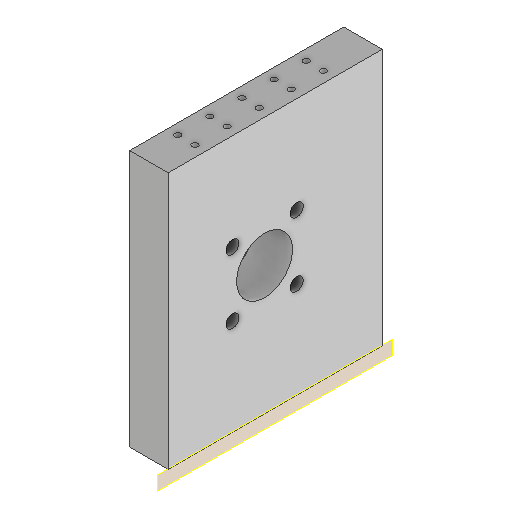
# Autodesk Inventor part: OpenFrameAdapter_2
Saved by Autodesk Inventor 2024.1 (Build 281209000, 209)
## iProperties
Created: 2024-06-05
Part Number: OpenFrameAdapter_2
Material: Generisch
Document SubType Name: Modeling
Designer: diederichbenedict
Density: 1 g/cm^3
Appearance: Vorgabe
Author: diederichbenedict
Autodesk Inventor part; units mm, degrees
ref_plane "YZ Plane" through (0, 0, 0) normal (1, 0, 0) x (0, 1, 0)
ref_plane "XZ Plane" through (0, 0, 0) normal (0, 1, 0) x (-1, 0, 0)
ref_plane "XY Plane" through (0, 0, 0) normal (0, 0, 1) x (1, 0, 0)
ref_plane "Arbeitsebene1" through (302.488, 50, 0) normal (1, 0, 0) x (0, -1, 0)
sketch "Skizze1" plane through (302.488, 50, 0) normal (1, 0, 0) x (0, -1, 0)
  line L0 (100, -120) -> (0, -120) projected
  line L1 (0, 0) -> (100, 0) projected
  line L2 (100, -120) -> (0, -120)
  line L3 (0, -120) -> (0, 0)
  line L4 (0, 0) -> (100, 0)
  line L5 (100, 0) -> (100, -120)
  circle A0 centre (55, -60) radius 13.0556 projected
  point P0 (50, 0)
  constraints: 8 end point, 2 parallel, 1 horizontal, 1 perpendicular
extrude "Extrusion1" add sketch "Skizze1" against normal blind 18
sketch "Skizze2" plane through (302.488, -50, 0) normal (0, 0, -1) x (-1, 0, 0)
  circle A0 centre (186.5, 89.5) radius 1.5 projected
  circle A1 centre (100.8, 89.5) radius 1.5 projected
  circle A2 centre (139.4003, 16.8597) radius 1.55 projected
  line L0 (398.9827, 14) -> (394.9827, 14) projected
  line L1 (394.9827, 14) -> (394.9827, 79) projected
  line L2 (394.9827, 79) -> (398.9827, 79) projected
  line L3 (398.9827, 79) -> (398.9827, 14) projected
  line L4 (252.25, 9) -> (252.25, 11.4) projected
  line L5 (252.25, 11.4) -> (257.75, 11.4) projected
  line L6 (257.75, 11.4) -> (257.75, 9) projected
  line L7 (257.75, 9) -> (252.25, 9) projected
  line L8 (457.75, 11.4) -> (457.75, 9) projected
  line L9 (457.75, 9) -> (452.25, 9) projected
  line L10 (452.25, 9) -> (452.25, 11.4) projected
  line L11 (452.25, 11.4) -> (457.75, 11.4) projected
  line L12 (57.75, 9) -> (52.25, 9) projected
  line L13 (52.25, 9) -> (52.25, 11.4) projected
  line L14 (52.25, 11.4) -> (57.75, 11.4) projected
  line L15 (57.75, 11.4) -> (57.75, 9) projected
  line L16 (352.25, 9) -> (352.25, 11.4) projected
  line L17 (352.25, 11.4) -> (357.75, 11.4) projected
  line L18 (357.75, 11.4) -> (357.75, 9) projected
  line L19 (357.75, 9) -> (352.25, 9) projected
  line L20 (157.75, 9) -> (152.25, 9) projected
  line L21 (152.25, 9) -> (152.25, 11.4) projected
  line L22 (152.25, 11.4) -> (157.75, 11.4) projected
  line L23 (157.75, 11.4) -> (157.75, 9) projected
  line L24 (257.75, 91) -> (257.75, 88.6) projected
  line L25 (257.75, 88.6) -> (252.25, 88.6) projected
  line L26 (252.25, 88.6) -> (252.25, 91) projected
  line L27 (252.25, 91) -> (257.75, 91) projected
  line L28 (157.75, 91) -> (157.75, 88.6) projected
  line L29 (157.75, 88.6) -> (152.25, 88.6) projected
  line L30 (152.25, 88.6) -> (152.25, 91) projected
  line L31 (152.25, 91) -> (157.75, 91) projected
  line L32 (357.75, 91) -> (357.75, 88.6) projected
  line L33 (357.75, 88.6) -> (352.25, 88.6) projected
  line L34 (352.25, 88.6) -> (352.25, 91) projected
  line L35 (352.25, 91) -> (357.75, 91) projected
  line L36 (57.75, 91) -> (57.75, 88.6) projected
  line L37 (57.75, 88.6) -> (52.25, 88.6) projected
  line L38 (52.25, 88.6) -> (52.25, 91) projected
  line L39 (52.25, 91) -> (57.75, 91) projected
  line L40 (452.25, 88.6) -> (452.25, 91) projected
  line L41 (452.25, 91) -> (457.75, 91) projected
  line L42 (457.75, 91) -> (457.75, 88.6) projected
  line L43 (457.75, 88.6) -> (452.25, 88.6) projected
  line L44 (449.9, 0) -> (449.9, 6) projected
  line L45 (449.9, 6) -> (460.1, 6) projected
  line L46 (460.1, 6) -> (460.1, 0) projected
  line L47 (460.1, 0) -> (490, 0) projected
  line L48 (490, 0) -> (490, 94) projected
  line L49 (490, 94) -> (470, 94) projected
  line L50 (470, 94) -> (470, 100) projected
  line L51 (470, 100) -> (460.1, 100) projected
  line L52 (460.1, 100) -> (460.1, 94) projected
  line L53 (460.1, 94) -> (449.9, 94) projected
  line L54 (449.9, 94) -> (449.9, 100) projected
  line L55 (449.9, 100) -> (440.1, 100) projected
  line L56 (440.1, 100) -> (440.1, 94) projected
  line L57 (440.1, 94) -> (429.9, 94) projected
  line L58 (429.9, 94) -> (429.9, 100) projected
  line L59 (429.9, 100) -> (420.1, 100) projected
  line L60 (420.1, 100) -> (420.1, 94) projected
  line L61 (420.1, 94) -> (409.9, 94) projected
  line L62 (409.9, 94) -> (409.9, 100) projected
  line L63 (409.9, 100) -> (400.1, 100) projected
  line L64 (400.1, 100) -> (400.1, 94) projected
  line L65 (400.1, 94) -> (389.9, 94) projected
  line L66 (389.9, 94) -> (389.9, 100) projected
  line L67 (389.9, 100) -> (380.1, 100) projected
  line L68 (380.1, 100) -> (380.1, 94) projected
  line L69 (380.1, 94) -> (369.9, 94) projected
  line L70 (369.9, 94) -> (369.9, 100) projected
  line L71 (369.9, 100) -> (360.1, 100) projected
  line L72 (360.1, 100) -> (360.1, 94) projected
  line L73 (360.1, 94) -> (349.9, 94) projected
  line L74 (349.9, 94) -> (349.9, 100) projected
  line L75 (349.9, 100) -> (340.1, 100) projected
  line L76 (340.1, 100) -> (340.1, 94) projected
  line L77 (340.1, 94) -> (329.9, 94) projected
  line L78 (329.9, 94) -> (329.9, 100) projected
  line L79 (329.9, 100) -> (320.1, 100) projected
  line L80 (320.1, 100) -> (320.1, 94) projected
  line L81 (320.1, 94) -> (309.9, 94) projected
  line L82 (309.9, 94) -> (309.9, 100) projected
  line L83 (309.9, 100) -> (300.1, 100) projected
  line L84 (300.1, 100) -> (300.1, 94) projected
  line L85 (300.1, 94) -> (289.9, 94) projected
  line L86 (289.9, 94) -> (289.9, 100) projected
  line L87 (289.9, 100) -> (280.1, 100) projected
  line L88 (280.1, 100) -> (280.1, 94) projected
  line L89 (280.1, 94) -> (269.9, 94) projected
  line L90 (269.9, 94) -> (269.9, 100) projected
  line L91 (269.9, 100) -> (260.1, 100) projected
  line L92 (260.1, 100) -> (260.1, 94) projected
  line L93 (260.1, 94) -> (249.9, 94) projected
  line L94 (249.9, 94) -> (249.9, 100) projected
  line L95 (249.9, 100) -> (240.1, 100) projected
  line L96 (240.1, 100) -> (240.1, 94) projected
  line L97 (240.1, 94) -> (229.9, 94) projected
  line L98 (229.9, 94) -> (229.9, 100) projected
  line L99 (229.9, 100) -> (220.1, 100) projected
  line L100 (220.1, 100) -> (220.1, 94) projected
  line L101 (220.1, 94) -> (209.9, 94) projected
  line L102 (209.9, 94) -> (209.9, 100) projected
  line L103 (209.9, 100) -> (200.1, 100) projected
  line L104 (200.1, 100) -> (200.1, 94) projected
  line L105 (200.1, 94) -> (189.9, 94) projected
  line L106 (189.9, 94) -> (189.9, 100) projected
  line L107 (189.9, 100) -> (180.1, 100) projected
  line L108 (180.1, 100) -> (180.1, 94) projected
  line L109 (180.1, 94) -> (169.9, 94) projected
  line L110 (169.9, 94) -> (169.9, 100) projected
  line L111 (169.9, 100) -> (160.1, 100) projected
  line L112 (160.1, 100) -> (160.1, 94) projected
  line L113 (160.1, 94) -> (149.9, 94) projected
  line L114 (149.9, 94) -> (149.9, 100) projected
  line L115 (149.9, 100) -> (140.1, 100) projected
  line L116 (140.1, 100) -> (140.1, 94) projected
  line L117 (140.1, 94) -> (129.9, 94) projected
  line L118 (129.9, 94) -> (129.9, 100) projected
  line L119 (129.9, 100) -> (120.1, 100) projected
  line L120 (120.1, 100) -> (120.1, 94) projected
  line L121 (120.1, 94) -> (109.9, 94) projected
  line L122 (109.9, 94) -> (109.9, 100) projected
  line L123 (109.9, 100) -> (100.1, 100) projected
  line L124 (100.1, 100) -> (100.1, 94) projected
  line L125 (100.1, 94) -> (89.9, 94) projected
  line L126 (89.9, 94) -> (89.9, 100) projected
  line L127 (89.9, 100) -> (80.1, 100) projected
  line L128 (80.1, 100) -> (80.1, 94) projected
  line L129 (80.1, 94) -> (69.9, 94) projected
  line L130 (69.9, 94) -> (69.9, 100) projected
  line L131 (69.9, 100) -> (60.1, 100) projected
  line L132 (60.1, 100) -> (60.1, 94) projected
  line L133 (60.1, 94) -> (49.9, 94) projected
  line L134 (49.9, 94) -> (49.9, 100) projected
  line L135 (49.9, 100) -> (0, 100) projected
  line L136 (0, 100) -> (0, 0) projected
  line L137 (0, 0) -> (49.9, 0) projected
  line L138 (49.9, 0) -> (49.9, 6) projected
  line L139 (49.9, 6) -> (60.1, 6) projected
  line L140 (60.1, 6) -> (60.1, 0) projected
  line L141 (60.1, 0) -> (69.9, 0) projected
  line L142 (69.9, 0) -> (69.9, 6) projected
  line L143 (69.9, 6) -> (80.1, 6) projected
  line L144 (80.1, 6) -> (80.1, 0) projected
  line L145 (80.1, 0) -> (89.9, 0) projected
  line L146 (89.9, 0) -> (89.9, 6) projected
  line L147 (89.9, 6) -> (100.1, 6) projected
  line L148 (100.1, 6) -> (100.1, 0) projected
  line L149 (100.1, 0) -> (109.9, 0) projected
  line L150 (109.9, 0) -> (109.9, 6) projected
  line L151 (109.9, 6) -> (120.1, 6) projected
  line L152 (120.1, 6) -> (120.1, 0) projected
  line L153 (120.1, 0) -> (129.9, 0) projected
  line L154 (129.9, 0) -> (129.9, 6) projected
  line L155 (129.9, 6) -> (140.1, 6) projected
  line L156 (140.1, 6) -> (140.1, 0) projected
  line L157 (140.1, 0) -> (149.9, 0) projected
  line L158 (149.9, 0) -> (149.9, 6) projected
  line L159 (149.9, 6) -> (160.1, 6) projected
  line L160 (160.1, 6) -> (160.1, 0) projected
  line L161 (160.1, 0) -> (169.9, 0) projected
  line L162 (169.9, 0) -> (169.9, 6) projected
  line L163 (169.9, 6) -> (180.1, 6) projected
  line L164 (180.1, 6) -> (180.1, 0) projected
  line L165 (180.1, 0) -> (189.9, 0) projected
  line L166 (189.9, 0) -> (189.9, 6) projected
  line L167 (189.9, 6) -> (200.1, 6) projected
  line L168 (200.1, 6) -> (200.1, 0) projected
  line L169 (200.1, 0) -> (209.9, 0) projected
  line L170 (209.9, 0) -> (209.9, 6) projected
  line L171 (209.9, 6) -> (220.1, 6) projected
  line L172 (220.1, 6) -> (220.1, 0) projected
  line L173 (220.1, 0) -> (229.9, 0) projected
  line L174 (229.9, 0) -> (229.9, 6) projected
  line L175 (229.9, 6) -> (240.1, 6) projected
  line L176 (240.1, 6) -> (240.1, 0) projected
  line L177 (240.1, 0) -> (249.9, 0) projected
  line L178 (249.9, 0) -> (249.9, 6) projected
  line L179 (249.9, 6) -> (260.1, 6) projected
  line L180 (260.1, 6) -> (260.1, 0) projected
  line L181 (260.1, 0) -> (269.9, 0) projected
  line L182 (269.9, 0) -> (269.9, 6) projected
  line L183 (269.9, 6) -> (280.1, 6) projected
  line L184 (280.1, 6) -> (280.1, 0) projected
  line L185 (280.1, 0) -> (289.9, 0) projected
  line L186 (289.9, 0) -> (289.9, 6) projected
  line L187 (289.9, 6) -> (300.1, 6) projected
  line L188 (300.1, 6) -> (300.1, 0) projected
  line L189 (300.1, 0) -> (309.9, 0) projected
  line L190 (309.9, 0) -> (309.9, 6) projected
  line L191 (309.9, 6) -> (320.1, 6) projected
  line L192 (320.1, 6) -> (320.1, 0) projected
  line L193 (320.1, 0) -> (329.9, 0) projected
  line L194 (329.9, 0) -> (329.9, 6) projected
  line L195 (329.9, 6) -> (340.1, 6) projected
  line L196 (340.1, 6) -> (340.1, 0) projected
  line L197 (340.1, 0) -> (349.9, 0) projected
  line L198 (349.9, 0) -> (349.9, 6) projected
  line L199 (349.9, 6) -> (360.1, 6) projected
  line L200 (360.1, 6) -> (360.1, 0) projected
  line L201 (360.1, 0) -> (369.9, 0) projected
  line L202 (369.9, 0) -> (369.9, 6) projected
  line L203 (369.9, 6) -> (380.1, 6) projected
  line L204 (380.1, 6) -> (380.1, 0) projected
  line L205 (380.1, 0) -> (389.9, 0) projected
  line L206 (389.9, 0) -> (389.9, 6) projected
  line L207 (389.9, 6) -> (400.1, 6) projected
  line L208 (400.1, 6) -> (400.1, 0) projected
  line L209 (400.1, 0) -> (409.9, 0) projected
  line L210 (409.9, 0) -> (409.9, 6) projected
  line L211 (409.9, 6) -> (420.1, 6) projected
  line L212 (420.1, 6) -> (420.1, 0) projected
  line L213 (420.1, 0) -> (429.9, 0) projected
  line L214 (429.9, 0) -> (429.9, 6) projected
  line L215 (429.9, 6) -> (440.1, 6) projected
  line L216 (440.1, 6) -> (440.1, 0) projected
  line L217 (440.1, 0) -> (449.9, 0) projected
  circle A3 centre (5, 47.5) radius 1.6 projected
  circle A4 centre (5, 62.5) radius 1.6 projected
  circle A5 centre (5, 32.5) radius 1.6 projected
  circle A6 centre (5, 77.5) radius 1.6 projected
  circle A7 centre (5, 17.5) radius 1.6 projected
  point P0 (302.488, 50)
hole "Bohrung1" at (297.488, -32.5, 0) at (297.488, -17.5, 0) at (297.488, -2.5, 0) at (297.488, 12.5, 0) at (297.488, 27.5, 0) direction (0, 0, 1) diameter 2.8 depth 14 tip angle 118
sketch "Skizze3" plane through (302.488, -50, 120) normal (0, 0, 1) x (1, 0, 0)
  circle A0 centre (-13.0375, 47.5) radius 1.6 projected
  circle A1 centre (-13.0375, 62.5) radius 1.6 projected
  circle A2 centre (-13.0375, 32.5) radius 1.6 projected
  circle A3 centre (-13.0375, 77.5) radius 1.6 projected
  circle A4 centre (-13.0375, 17.5) radius 1.6 projected
  line L0 (-97.75, 88.6) -> (-97.75, 91) projected
  line L1 (-97.75, 91) -> (-92.25, 91) projected
  line L2 (-92.25, 91) -> (-92.25, 88.6) projected
  line L3 (-92.25, 88.6) -> (-97.75, 88.6) projected
  line L4 (-57.75, 88.6) -> (-57.75, 91) projected
  line L5 (-57.75, 91) -> (-52.25, 91) projected
  line L6 (-52.25, 91) -> (-52.25, 88.6) projected
  line L7 (-52.25, 88.6) -> (-57.75, 88.6) projected
  line L8 (-100.2875, 11.4) -> (-100.2875, 9) projected
  line L9 (-100.2875, 9) -> (-105.7875, 9) projected
  line L10 (-105.7875, 9) -> (-105.7875, 11.4) projected
  line L11 (-105.7875, 11.4) -> (-100.2875, 11.4) projected
  line L12 (-25.7875, 9) -> (-25.7875, 11.4) projected
  line L13 (-25.7875, 11.4) -> (-20.2875, 11.4) projected
  line L14 (-20.2875, 11.4) -> (-20.2875, 9) projected
  line L15 (-20.2875, 9) -> (-25.7875, 9) projected
  line L16 (-123.0375, 8) -> (-122.8375, 8) projected
  line L17 (-122.8375, 8) -> (-122.8375, 6) projected
  line L18 (-123.0375, 6) -> (-123.0375, 3.8071) projected
  line L19 (-120.1, 6) -> (-109.9, 6) projected
  line L20 (-109.9, 6) -> (-117.9375, 0) projected
  line L21 (-117.9375, 0) -> (-108.1375, 0) projected
  line L22 (-108.1375, 0) -> (-100.1, 6) projected
  line L23 (-100.1, 6) -> (-89.9, 6) projected
  line L24 (-89.9, 6) -> (-97.9375, 0) projected
  line L25 (-97.9375, 0) -> (-88.1375, 0) projected
  line L26 (-88.1375, 0) -> (-80.1, 6) projected
  line L27 (-80.1, 6) -> (-69.9, 6) projected
  line L28 (-69.9, 6) -> (-77.9375, 0) projected
  line L29 (-77.9375, 0) -> (-68.1375, 0) projected
  line L30 (-68.1375, 0) -> (-60.1, 6) projected
  line L31 (-60.1, 6) -> (-49.9, 6) projected
  line L32 (-49.9, 6) -> (-57.9375, 0) projected
  line L33 (-57.9375, 0) -> (-48.1375, 0) projected
  line L34 (-48.1375, 0) -> (-40.1, 6) projected
  line L35 (-40.1, 6) -> (-29.9, 6) projected
  line L36 (-29.9, 6) -> (-37.9375, 0) projected
  line L37 (-37.9375, 0) -> (-28.1375, 0) projected
  line L38 (-28.1375, 0) -> (-20.1, 6) projected
  line L39 (-20.1, 6) -> (-9.9, 6) projected
  line L40 (-9.9, 6) -> (-17.9375, 0) projected
  line L41 (-17.9375, 0) -> (-8.0375, 0) projected
  line L42 (-49.9, 100) -> (-49.9, 94) projected
  line L43 (-49.9, 94) -> (-60.1, 94) projected
  line L44 (-60.1, 94) -> (-60.1, 100) projected
  line L45 (-69.9, 100) -> (-69.9, 94) projected
  line L46 (-69.9, 94) -> (-80.1, 94) projected
  line L47 (-80.1, 94) -> (-80.1, 100) projected
  line L48 (-89.9, 100) -> (-89.9, 94) projected
  line L49 (-89.9, 94) -> (-100.1, 94) projected
  line L50 (-100.1, 94) -> (-100.1, 100) projected
  line L51 (-110, 100) -> (-110, 94) projected
  line L52 (-110, 94) -> (-115, 94) projected
  circle A5 centre (-5, 77.5) radius 1.4 projected
  circle A6 centre (-5, 62.5) radius 1.4 projected
  circle A7 centre (-5, 47.5) radius 1.4 projected
  circle A8 centre (-5, 32.5) radius 1.4 projected
  circle A9 centre (-5, 17.5) radius 1.4 projected
  line L53 (0, 0) -> (0, 100) projected
  line L54 (0, 0) -> (-18, 0) projected
  line L55 (-18, 100) -> (-18, 0) projected
  line L56 (0, 100) -> (-18, 100) projected
  line L57 (-122.8375, 6) -> (-123.0375, 6) projected
  line L58 (-123.0375, 3.8071) -> (-120.1, 6) projected
  line L59 (-8.0375, 0) -> (-8.0375, 100) projected
  line L60 (-8.0375, 100) -> (-49.9, 100) projected
  line L61 (-60.1, 100) -> (-69.9, 100) projected
  line L62 (-80.1, 100) -> (-89.9, 100) projected
  line L63 (-100.1, 100) -> (-110, 100) projected
  line L64 (-115, 94) -> (-115, 100) projected
  line L65 (-115, 100) -> (-123.0375, 100) projected
  line L66 (-123.0375, 100) -> (-123.0375, 8) projected
  point P0 (-302.488, 50)
hole "Bohrung2" at (289.4504, 27.5, 120) at (289.4504, 12.5, 120) at (289.4504, -2.5, 120) at (289.4504, -17.5, 120) at (289.4504, -32.5, 120) at (297.488, -32.5, 120) at (297.488, -17.5, 120) at (297.488, -2.5, 120) at (297.488, 12.5, 120) at (297.488, 27.5, 120) direction (0, 0, -1) diameter 2.8 depth 14 tip angle 118
sketch "Skizze4" plane through (284.488, 50, 0) normal (-1, 0, 0) x (0, 0, 1)
  line L0 (39.934, -37.0712) -> (39.934, -72.9288) projected
  line L1 (39.934, -72.9288) -> (42.0712, -75.066) projected
  line L2 (42.0712, -75.066) -> (77.9288, -75.066) projected
  line L3 (77.9288, -75.066) -> (80.066, -72.9288) projected
  line L4 (80.066, -72.9288) -> (80.066, -37.0712) projected
  line L5 (80.066, -37.0712) -> (77.9288, -34.934) projected
  line L6 (77.9288, -34.934) -> (42.0712, -34.934) projected
  line L7 (42.0712, -34.934) -> (39.934, -37.0712) projected
  circle A0 centre (75, -70) radius 3.2639 projected
  circle A1 centre (45, -70) radius 3.2639 projected
  circle A2 centre (75, -40) radius 3.2639 projected
  circle A3 centre (45, -40) radius 3.2639 projected
  circle A4 centre (60, -55) radius 13.3985 projected
  point P0 (0, -50)
hole "Bohrung3" at (284.488, -20, 75) at (284.488, -20, 45) at (284.488, 10, 45) at (284.488, 10, 75) direction (1, 0, 0) diameter 6.1 end through all
